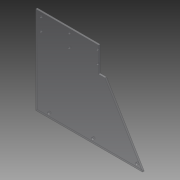
# Autodesk Inventor part: Hopper Right Side Leg
Saved by Autodesk Inventor 2014 SP1 (Build 180222100, 222)
## iProperties
Created: 2013-12-16
Part Number: Hopper Right Side Leg
Material: Polycarbonate, Clear
Document SubType Name: Modeling
Designer: Moses
Mass: 110.326 g
Surface Area: 605.317 cm^2
Volume: 91.9384 cm^3
Density: 1.2 g/cm^3
Appearance: Polycarbonate - Clear
Author: Moses
Autodesk Inventor part; units mm, degrees
ref_plane "YZ Plane" through (0, 0, 0) normal (1, 0, 0) x (0, 1, 0)
ref_plane "XZ Plane" through (0, 0, 0) normal (0, 1, 0) x (-1, 0, 0)
ref_plane "XY Plane" through (0, 0, 0) normal (0, 0, 1) x (1, 0, 0)
sketch "Sketch1" plane through (0, 0, 0) normal (0, 0, 1) x (1, 0, 0)
  line L0 (0, 177.8) -> (0, 0)
  line L1 (0, 0) -> (215.9, 0)
  line L2 (0, 177.8) -> (127, 177.8)
  line L3 (127, 177.8) -> (127, 127)
  circle A0 centre (9.525, 168.275) radius 1.5875
  circle A1 centre (66.675, 168.275) radius 1.5875
  circle A2 centre (123.825, 168.275) radius 1.5875
  circle A3 centre (9.525, 142.875) radius 1.5875
  circle A4 centre (66.675, 142.875) radius 1.5875
  circle A5 centre (123.825, 142.875) radius 1.5875
  line L4 (127, 127) -> (139.7, 127)
  line L5 (139.7, 127) -> (215.9, 0)
  circle A6 centre (114.3, 7.5406) radius 1.7145 projected
  circle A7 centre (25.4, 7.5406) radius 1.7145 projected
  circle A8 centre (203.2, 7.5406) radius 1.7145 projected
  line L6 (0, -0.7937) -> (0, 15.0812) construction
  line L7 (0, -0.7937) -> (215.9, -0.7938) construction
  line L8 (215.9, 15.0812) -> (215.9, -0.7938) construction
  line L9 (0, 15.0812) -> (215.9, 15.0812) construction
  dimension "d0" = 177.8
  dimension "d1" = 215.9
  dimension "d2" = 127
  dimension "d3" = 50.8
  dimension "d7" = 3.175
  dimension "d10" = 57.15
  dimension "d13" = 25.4
  dimension "d16" = 9.525
  dimension "d17" = 9.525
  dimension "d18" = 12.7
  constraints: 12 end point, 6 centre point, 2 horizontal, 2 perpendicular, 2 vertical, 1 coincident, 1 parallel, 10 other
  measures "d0" distance of L0.start L0.end
  measures "d1" distance of L0.end L1.end
  measures "d2" distance of L0.start L2.end
  measures "d3" distance of L2.end L3.end
  measures "d7" diameter of A0
  measures "d10" distance of A0.centre A1.centre
  measures "d13" distance of A0.centre A3.centre
  measures "d16" distance from line of A0.centre L0
  measures "d17" distance from line of L2 A0.centre
  measures "d18" distance of L3.end L4.end
extrude "Extrusion1" add sketch "Sketch1" along normal blind 3.175
body "Solid1"
